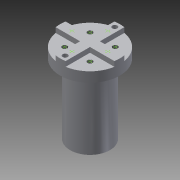
# Autodesk Inventor part: Achse
Saved by Autodesk Inventor 2013 (Build 170138000, 138)
## iProperties
Created: 2012-12-21
Part Number: Achse
Material: Aluminium 6061
Document SubType Name: Modeling
Designer: Lukas
Density: 1 g/cm^3
Author: Lukas
Autodesk Inventor part; units mm, degrees
ref_plane "YZ Plane" through (0, 0, 0) normal (1, 0, 0) x (0, 1, 0)
ref_plane "XZ Plane" through (0, 0, 0) normal (0, 1, 0) x (-1, 0, 0)
ref_plane "XY Plane" through (0, 0, 0) normal (0, 0, 1) x (1, 0, 0)
sketch "Skizze1" plane through (0, 0, 0) normal (1, 0, 0) x (0, 1, 0)
  line L0 (20, 20) -> (0, 20)
  line L1 (0, 20) -> (20, 20)
  line L2 (20, 20) -> (20, 90)
  line L3 (20, 90) -> (0, 90)
  line L4 (0, 90) -> (0, 20)
  line L5 (0, 90) -> (30, 90)
  line L6 (30, 90) -> (30, 100)
  line L7 (30, 100) -> (0, 100)
  line L8 (0, 100) -> (0, 90)
  dimension "d0" = 20
  dimension "d2" = 20
  dimension "d3" = 70
  dimension "d4" = 30
  dimension "d5" = 10
  constraints: 18 end point, 4 parallel, 2 horizontal, 2 perpendicular
  measures "d0" distance of L0.end L0.start
  measures "d2" distance of L3.end L2.end
  measures "d3" distance of L2.end L1.end
  measures "d4" distance of L7.end L6.end
  measures "d5" distance of L6.end L5.end
revolve "Umdrehung1" add sketch "Skizze1" angle 360 about axis through (0, 0, 90) along (0, 0, -1)
sketch "Skizze5" plane through (0, 0, 100) normal (0, 0, 1) x (1, 0, 0)
  circle A0 centre (0, 0) radius 30 projected
  line L0 (5, 5) -> (29.5804, 5)
  line L1 (5, -5) -> (29.5804, -5)
  line L2 (5, -5) -> (5, -29.5804)
  line L3 (5, 5) -> (5, 29.5804)
  line L4 (-5, 5) -> (-5, 29.5804)
  line L5 (-5, 5) -> (-29.5804, 5)
  line L6 (-5, -5) -> (-29.5804, -5)
  line L7 (-5, -5) -> (-5, -29.5804)
  arc A1 (5, 29.5804) -> (-5, 29.5804) centre (0, 0) ccw
  arc A2 (29.5804, -5) -> (29.5804, 5) centre (0, 0) ccw
  arc A3 (-5, -29.5804) -> (5, -29.5804) centre (0, 0) ccw
  arc A4 (-29.5804, 5) -> (-29.5804, -5) centre (0, 0) ccw
  constraints: 16 end point, 8 point on circle, 4 centre point, 4 coincident, 3 equal length, 3 perpendicular, 1 horizontal, 10 other
extrude "Extrusion3" add sketch "Skizze5" along normal blind 5 contours A0 L1 L2 L7 L6 L5 L4 L3 L0
sketch "Skizze8" plane through (5, -5, 100) normal (0, 0, 1) x (1, 0, 0)
  arc A0 (0, -24.5804) -> (24.5804, 0) centre (-5, 5) ccw projected
  circle A1 centre (-5, 5) radius 18
  line L0 (-5, 5) -> (7.7279, 17.7279)
  line L1 (-5, 5) -> (13, 5) construction
  line L2 (-5, 5) -> (7.7279, -7.7279)
  line L3 (-5, 5) -> (-17.7279, -7.7279)
  line L4 (-5, 5) -> (-17.7279, 17.7279)
  dimension "d33" = 36
  dimension "d34" = 45
  constraints: 10 end point, 5 coincident, 4 point on circle, 3 perpendicular, 1 centre point, 1 equal length, 1 horizontal
  measures "d33" diameter of A1
  measures "d34" angle of L1 L0
hole "Bohrung2" at (-12.7279, -12.7279, 100) at (12.7279, -12.7279, 100) at (12.7279, 12.7279, 100) at (-12.7279, 12.7279, 100) direction (0, 0, -1) diameter 5 depth 8 tip angle 118
thread "Gewinde1" size "M5x0.8" class "6H" standard "ANSI Metric M Profile" full length
thread "Gewinde3" size "M5x0.8" class "6H" standard "ANSI Metric M Profile" full length
thread "Gewinde5" size "M5x0.8" class "6H" standard "ANSI Metric M Profile" full length
thread "Gewinde7" size "M5x0.8" class "6H" standard "ANSI Metric M Profile" full length
sketch "Skizze16" plane through (0, 0, 105) normal (0, 0, 1) x (1, 0, 0)
  arc A0 (5, 29.5804) -> (-5, 29.5804) centre (0, 0) ccw projected
  point P0 (0, -25)
  point P1 (0, 25)
  dimension "d125" = 25
  dimension "d126" = 25
  measures "d125" distance of point (0, 25) A0.centre
  measures "d126" distance of A0.centre point (0, -25)
hole "Bohrung16" at (0, -25, 105) at (0, 25, 105) direction (0, 0, -1) diameter 5 end through all
sketch "Skizze9" plane through (0, 0, 105) normal (0, 0, 1) x (1, 0, 0)
  point P0 (0, 18)
  point P1 (-18, 0)
  point P2 (0, -18)
  point P3 (18, 0)
sketch "Skizze10" plane through (5, -5, 100) normal (0, 0, 1) x (1, 0, 0)
  point P0 (7.7279, 17.7279)
  point P1 (-17.7279, 17.7279)
  point P2 (-17.7279, -7.7279)
  point P3 (7.7279, -7.7279)
  point P4 (-17.7279, -7.7279)
sketch "Skizze11" plane through (5, -5, 100) normal (0, 0, 1) x (1, 0, 0)
  point P0 (7.7279, 17.7279)
  point P1 (-17.7279, 17.7279)
  point P2 (-17.7279, -7.7279)
  point P3 (7.7279, -7.7279)
  point P4 (-17.7279, -7.7279)
sketch "Skizze12" plane through (0, 0, 105) normal (0, 0, 1) x (1, 0, 0)
  point P0 (0, 18)
  point P1 (-18, 0)
  point P2 (0, -18)
  point P3 (18, 0)
sketch "Skizze14" plane through (5, 5, 100) normal (0, 0, 1) x (1, 0, 0)
  point P0 (-5, 13)
  point P1 (-23, -5)
  point P2 (-5, -23)
  point P3 (13, -5)
sketch "Skizze15" plane through (-29.5804, 5, 100) normal (0, 0, 1) x (1, 0, 0)
  point P0 (42.3083, 7.7279)
  point P1 (16.8525, 7.7279)
  point P2 (16.8525, -17.7279)
  point P3 (42.3083, -17.7279)
  point P4 (16.8525, -17.7279)
sketch "Skizze17" plane through (-29.5804, -5, 100) normal (0, 0, 1) x (1, 0, 0)
  point P0 (42.3083, 17.7279)
  point P1 (16.8525, 17.7279)
  point P2 (16.8525, -7.7279)
  point P3 (42.3083, -7.7279)
hole "Bohrung17" at (12.7279, 12.7279, 100) at (-12.7279, 12.7279, 100) at (-12.7279, -12.7279, 100) at (12.7279, -12.7279, 100) direction (0, 0, -1) diameter 4.134 depth 8.9618 tip angle 120 thread size "M5x0.8" class "6H" standard "ISO Metric profile"
